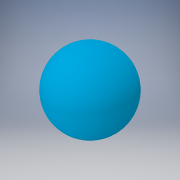
# Autodesk Inventor part: Ball
Saved by Autodesk Inventor 2018 (Build 220112000, 112)
## iProperties
Created: 2019-03-05
Part Number: Ball
Material: Generisch
Document SubType Name: Modeling
Designer: RedBots
Appearance: Himmelblau - mittel
Surface Area: 172.034 cm^2
Volume: 212.175 cm^3
Author: RedBots
Autodesk Inventor part; units mm, degrees
ref_plane "YZ Plane" through (0, 0, 0) normal (1, 0, 0) x (0, 1, 0)
ref_plane "XZ Plane" through (0, 0, 0) normal (0, 1, 0) x (-1, 0, 0)
ref_plane "XY Plane" through (0, 0, 0) normal (0, 0, 1) x (1, 0, 0)
sketch "Skizze1" plane through (0, 0, 0) normal (0, 0, 1) x (1, 0, 0)
  circle A0 centre (0, 0) radius 37
  line L0 (37, 0) -> (-37, 0)
  line L1 (-51.8, 0) -> (51.8, 0) projected
  dimension "d0" = 74
  dimension "d1" = 74
  constraints: 2 end point, 2 point on circle, 1 centre point, 1 coincident, 1 horizontal
  measures "d0" diameter of A0
  measures "d1" distance of L0.start L0.end
revolve "Umdrehung1" add sketch "Skizze1" angle 360 about axis through (-10, 0, 0) along (1, 0, 0) picked at (-11.1119, -5.3512) contours A0 L0
